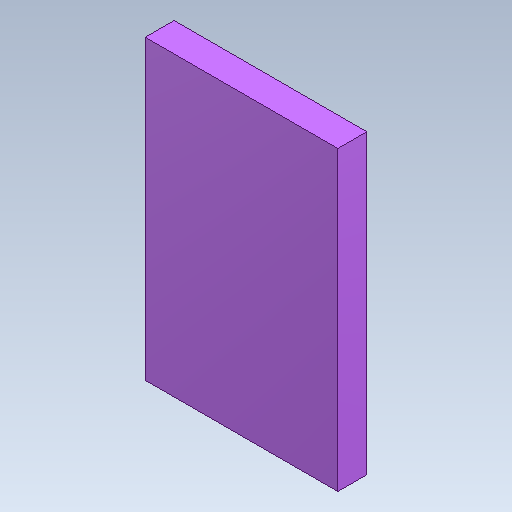
# Autodesk Inventor part: 7805DT
Saved by Autodesk Inventor 2020 (Build 240168000, 168)
## iProperties
Created: 2019-08-29
Part Number: 7805DT
Material: Generic
Document SubType Name: Modeling
Designer: psrob
Density: 1 g/cm^3
Appearance: TO252, 7805DT
Author: psrob
Autodesk Inventor part; units mm, degrees
ref_plane "YZ Plane" through (0, 0, 0) normal (1, 0, 0) x (0, 1, 0)
ref_plane "XZ Plane" through (0, 0, 0) normal (0, 1, 0) x (-1, 0, 0)
ref_plane "XY Plane" through (0, 0, 0) normal (0, 0, 1) x (1, 0, 0)
sketch "TO252, 7805DT_22" plane through (0, 0, 0) normal (0, 0, 1) x (1, 0, 0)
  line L0 (-3.277, 5.1054) -> (3.3786, 5.1054)
  line L1 (3.3786, 5.1054) -> (3.3786, -5.1562)
  line L2 (3.3786, -5.1562) -> (-3.277, -5.1562)
  line L3 (-3.277, -5.1562) -> (-3.277, 5.1054)
  constraints: 8 end point
extrude "Extrusion1" add sketch "TO252, 7805DT_22" along normal blind 1
body "Solid1"
